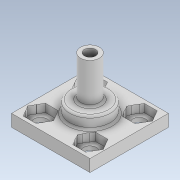
# Autodesk Inventor part: INTERFACE_MANIFOLD
Saved by Autodesk Inventor 2020 (Build 240168000, 168)
## iProperties
Created: 2020-07-07
Part Number: INTERFACE_MANIFOLD
Material: Generic
Document SubType Name: Modeling
Designer: Admin
Density: 1 g/cm^3
Appearance: Default
Author: Admin
Autodesk Inventor part; units mm, degrees
ref_plane "YZ Plane" through (0, 0, 0) normal (1, 0, 0) x (0, 1, 0)
ref_plane "XZ Plane" through (0, 0, 0) normal (0, 1, 0) x (-1, 0, 0)
ref_plane "XY Plane" through (0, 0, 0) normal (0, 0, 1) x (1, 0, 0)
sketch "Sketch1" plane through (0, 0, 0) normal (0, 1, 0) x (-1, 0, 0)
  line L0 (0, 0) -> (19.4, 0)
  line L1 (19.4, 0) -> (19.4, -19.4)
  line L2 (19.4, -19.4) -> (0, -19.4)
  line L3 (0, -19.4) -> (0, 0)
  dimension "d0" = 19.4
  dimension "d1" = 19.4
  constraints: 8 end point, 2 parallel, 1 horizontal, 1 perpendicular
  measures "d0" distance of L0.start L0.end
  measures "d1" distance of L2.end L0.start
extrude "Extrusion1" add sketch "Sketch1" along normal blind 3
sketch "Sketch2" plane through (0, 3, 0) normal (0, 1, 0) x (1, 0, 0)
  circle A0 centre (-15.8, 3.6) radius 1.6
  line L0 (-19.4, 19.4) -> (-19.4, 0) projected
  line L1 (-19.4, 0) -> (0, 0) projected
  dimension "d4" = 3.2
  dimension "d5" = 3.6
  dimension "d6" = 3.6
  constraints: 1 centre point
  measures "d4" diameter of A0
  measures "d5" distance from line of L0 A0.centre
  measures "d6" distance from line of L1 A0.centre
extrude "Extrusion2" cut sketch "Sketch2" against normal through all
pattern_linear "Rectangular Pattern1" count 2 spacing 12.2 along (0, 0, -1) count 2 spacing 12.2 along (1, 0, 0) of "Extrusion2"
sketch "Sketch3" plane through (0, 3, 0) normal (0, 1, 0) x (1, 0, 0)
  circle A0 centre (-9.7, 9.7) radius 5
  line L0 (-19.4, 0) -> (0, 0) projected
  line L1 (0, 0) -> (0, 19.4) projected
  dimension "d15" = 10
  dimension "d16" = 9.7
  dimension "d17" = 9.7
  constraints: 1 centre point
  measures "d15" diameter of A0
  measures "d16" distance from line of L0 A0.centre
  measures "d17" distance from line of L1 A0.centre
extrude "Extrusion3" add sketch "Sketch3" along normal blind 3
sketch "Sketch4" plane through (-9.7, 6, -9.7) normal (0, 1, 0) x (1, 0, 0)
  circle A0 centre (0, 0) radius 2.35
  line L0 (9.7, -9.7) -> (9.7, 9.7) projected
  line L1 (-9.7, -9.7) -> (9.7, -9.7) projected
  dimension "d20" = 4.7
  dimension "d21" = 9.7
  dimension "d22" = 9.7
  constraints: 1 centre point
  measures "d20" diameter of A0
  measures "d21" distance from line of L0 A0.centre
  measures "d22" distance from line of L1 A0.centre
extrude "Extrusion4" add sketch "Sketch4" along normal blind 10
fillet "Fillet1" radius 0.5 1 edges at (-14.7, 3, -9.7)
fillet "Fillet2" radius 0.5 1 edges at (-14.7, 6, -9.7)
fillet "Fillet3" radius 0.5 1 edges at (-12.05, 6, -9.7)
sketch "Sketch5" plane through (-9.7, 16, -9.7) normal (0, 1, 0) x (1, 0, 0)
  circle A0 centre (0, 0) radius 1.4
  line L0 (9.7, -9.7) -> (9.7, 9.7) projected
  line L1 (-9.7, -9.7) -> (9.7, -9.7) projected
  dimension "d28" = 2.8
  dimension "d29" = 9.7
  dimension "d30" = 9.7
  constraints: 1 centre point
  measures "d28" diameter of A0
  measures "d29" distance from line of L0 A0.centre
  measures "d30" distance from line of L1 A0.centre
extrude "Extrusion5" cut sketch "Sketch5" against normal through all
sketch "Sketch6" plane through (0, 3, 0) normal (0, 1, 0) x (1, 0, 0)
  circle A0 centre (-3.6, 3.6) radius 2.75
  line L0 (0, 0) -> (0, 19.4) projected
  line L1 (-19.4, 0) -> (0, 0) projected
  dimension "d33" = 5.5
  dimension "d34" = 3.6
  dimension "d35" = 3.6
  constraints: 1 centre point
  measures "d33" diameter of A0
  measures "d34" distance from line of L0 A0.centre
  measures "d35" distance from line of L1 A0.centre
extrude "Extrusion6" cut sketch "Sketch6" against normal blind 2
pattern_linear "Rectangular Pattern2" count 2 spacing 12.2 along (0, 0, -1) count 2 spacing 12.2 along (-1, 0, 0) of "Extrusion6"
sketch "Sketch7" plane through (0, 3, 0) normal (0, 1, 0) x (1, 0, 0)
  line L0 (-17.387, 18.55) -> (-14.2116, 18.55)
  line L1 (-14.2116, 18.55) -> (-12.6239, 15.8)
  line L2 (-12.6239, 15.8) -> (-14.2116, 13.05)
  line L3 (-14.2116, 13.05) -> (-17.387, 13.05)
  line L4 (-17.387, 13.05) -> (-18.9747, 15.8)
  line L5 (-18.9747, 15.8) -> (-17.387, 18.55)
  line L6 (-19.4, 19.4) -> (-19.4, 0) projected
  line L7 (0, 19.4) -> (-19.4, 19.4) projected
  point P0 (0, 0)
  dimension "d56" = 0
  dimension "d57" = 0
  dimension "d58" = 0
  dimension "d59" = 5.5
  dimension "d60" = 5.5
  dimension "d61" = 120
  dimension "d62" = 2.013
  dimension "d63" = 0.85
  constraints: 12 end point, 3 parallel, 1 horizontal
  measures "d56" vertical distance of L4.end L1.end
  measures "d57" horizontal distance of L0.start L3.end
  measures "d58" horizontal distance of L2.end L0.end
  measures "d59" distance between parallel lines of L3 L0
  measures "d60" distance between parallel lines of L4 L1
  measures "d61" angle of L5 L0
  measures "d62" distance from line of L0.start L6
  measures "d63" distance from line of L7 L0.start
extrude "Extrusion7" cut sketch "Sketch7" against normal blind 2
pattern_linear "Rectangular Pattern3" count 2 spacing 12.3 along (1, 0, 0) count 2 spacing 12.2 along (0, 0, 1) of "Extrusion7"
equation "\"d1\" = d0"
equation "\"d17\" = d16"
body "Solid1"
